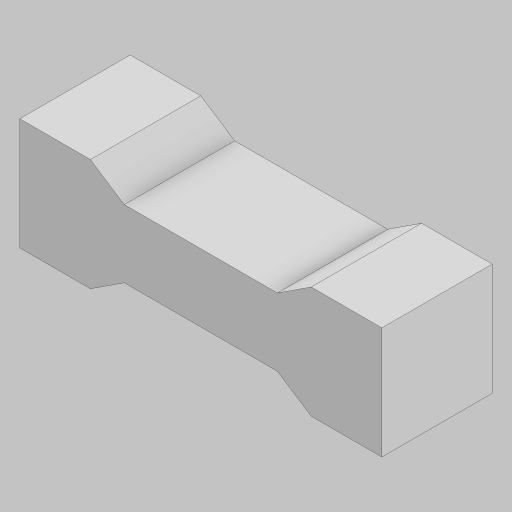
# Autodesk Inventor part: Spline_parametrizado
Saved by Autodesk Inventor 2023 (Build 270158000, 158)
## iProperties
Created: 2026-02-22
Part Number: Spline_parametrizado
Material: Genérico
Document SubType Name: Modeling
Designer: MARTIN MAESTRE
Density: 1 g/cm^3
Appearance: Valor por defecto
Author: MARTIN MAESTRE
Autodesk Inventor part; units mm, degrees
ref_plane "YZ Plane" through (0, 0, 0) normal (1, 0, 0) x (0, 1, 0)
ref_plane "XZ Plane" through (0, 0, 0) normal (0, 1, 0) x (-1, 0, 0)
ref_plane "XY Plane" through (0, 0, 0) normal (0, 0, 1) x (1, 0, 0)
sketch "Boceto1" plane through (0, 0, 0) normal (0, 0, 1) x (1, 0, 0)
  line L0 (0, 0) -> (0, 15.2)
  line L1 (0, 15.2) -> (9.6, 15.2)
  line L2 (0, 0) -> (9.6, 0)
  line L3 (9.6, 0) -> (14.6, 0) construction
  line L4 (14.6, 0) -> (24.6, 0) construction
  line L5 (24.6, 0) -> (24.6, 3) construction
  line L6 (24.6, 3) -> (14.2, 3)
  line L7 (14.2, 3) -> (9.6, 0)
  line L8 (24.6, 3) -> (24.6, 12.2)
  line L9 (24.6, 12.2) -> (14.2, 12.2)
  line L10 (14.2, 12.2) -> (9.6, 15.2)
  line L11 (49.2, 0) -> (49.2, 15.2)
  line L12 (49.2, 15.2) -> (39.6, 15.2)
  line L13 (49.2, 0) -> (39.6, 0)
  line L14 (39.6, 0) -> (34.6, 0) construction
  line L15 (34.6, 0) -> (24.6, 0) construction
  line L16 (24.6, 3) -> (35, 3)
  line L17 (35, 3) -> (39.6, 0)
  line L18 (24.6, 12.2) -> (35, 12.2)
  line L19 (35, 12.2) -> (39.6, 15.2)
  dimension "d0" = 15.2
  dimension "d1" = 9.6
  dimension "d2" = 9.6
  dimension "d3" = 5
  dimension "d4" = 10
  dimension "d5" = 3
  dimension "d6" = 10.4
  dimension "d7" = 9.2
  dimension "d8" = 10.4
  constraints: 40 end point, 7 symmetric about line, 5 horizontal, 2 perpendicular, 2 vertical
  measures "d0" distance of L0.start L0.end
  measures "d1" distance of L0.end L1.end
  measures "d2" distance of L0.start L2.end
  measures "d3" distance of L2.end L3.end
  measures "d4" distance of L3.end L4.end
  measures "d5" distance of L4.end L5.end
  measures "d6" distance of L5.end L6.end
  measures "d7" distance of L5.end L8.end
  measures "d8" distance of L8.end L9.end
extrude "Extrusión1" add sketch "Boceto1" along normal blind 15
equation "\"d4\" = Largo_seccion"
equation "\"d5\" = Espesor_centro"
equation "\"Largo_seccion\" = 10"
equation "\"Espesor_centro\" = 3"
